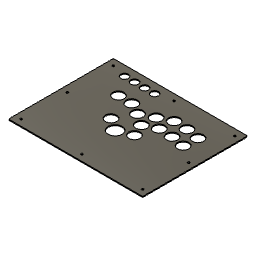
panel (Autodesk Fusion 360 design; units mm, degrees)
Autodesk Fusion 360 part; units mm, degrees
sketch "panel" plane through (0, 0, 0) normal (0, 0, 1) x (1, 0, 0)
  line L0 (62.8541, 263.5001) -> (357.1459, 263.5001)
  line L1 (357.1459, 263.5001) -> (357.1459, 33.5001)
  line L2 (357.1459, 33.5001) -> (62.8541, 33.5001)
  line L3 (62.8541, 33.5001) -> (62.8541, 263.5001)
  line L4 (137.8887, 199.6854) -> (139.7122, 197.8619)
  line L5 (139.7122, 199.6854) -> (137.8887, 197.8619)
  line L6 (167.3878, 199.4554) -> (169.2113, 197.6319)
  line L7 (169.2113, 199.4554) -> (167.3878, 197.6319)
  line L8 (193.5289, 185.7844) -> (195.3524, 183.9609)
  line L9 (195.3524, 185.7844) -> (193.5289, 183.9609)
  line L10 (220.9942, 199.2964) -> (222.8177, 197.4729)
  line L11 (222.8177, 199.2964) -> (220.9942, 197.4729)
  line L12 (247.5472, 212.1984) -> (249.3707, 210.3749)
  line L13 (249.3707, 212.1984) -> (247.5472, 210.3749)
  line L14 (277.0202, 210.8714) -> (278.8437, 209.0479)
  line L15 (278.8437, 210.8714) -> (277.0202, 209.0479)
  line L16 (306.1132, 205.9884) -> (307.9366, 204.1649)
  line L17 (307.9366, 205.9884) -> (306.1132, 204.1649)
  line L18 (304.0832, 175.4464) -> (305.9067, 173.6229)
  line L19 (305.9067, 175.4464) -> (304.0832, 173.6229)
  line L20 (274.9902, 180.3294) -> (276.8136, 178.5059)
  line L21 (276.8136, 180.3294) -> (274.9902, 178.5059)
  line L22 (245.5172, 181.6564) -> (247.3407, 179.8329)
  line L23 (247.3407, 181.6564) -> (245.5172, 179.8329)
  line L24 (218.9642, 168.7544) -> (220.7877, 166.9309)
  line L25 (220.7877, 168.7544) -> (218.9642, 166.9309)
  line L26 (230.8722, 141.9414) -> (232.6957, 140.1179)
  line L27 (232.6957, 141.9414) -> (230.8722, 140.1179)
  line L28 (173.1491, 148.1874) -> (174.9726, 146.3639)
  line L29 (174.9726, 148.1874) -> (173.1491, 146.3639)
  line L30 (200.3572, 129.9534) -> (202.1807, 128.1299)
  line L31 (202.1807, 129.9534) -> (200.3572, 128.1299)
  line L32 (108.0433, 242.9744) -> (109.8668, 241.1509)
  line L33 (109.8668, 242.9744) -> (108.0433, 241.1509)
  line L34 (130.0434, 242.9744) -> (131.8669, 241.1509)
  line L35 (131.8668, 242.9744) -> (130.0434, 241.1509)
  line L36 (152.0434, 242.9744) -> (153.8668, 241.1509)
  line L37 (153.8668, 242.9744) -> (152.0434, 241.1509)
  line L38 (174.0434, 242.9744) -> (175.8668, 241.1509)
  line L39 (175.8668, 242.9744) -> (174.0434, 241.1509)
  line L40 (75.8193, 250.5344) -> (77.6428, 248.7109)
  line L41 (77.6428, 250.5344) -> (75.8193, 248.7109)
  line L42 (75.8428, 149.3114) -> (77.6663, 147.4879)
  line L43 (77.6663, 149.3114) -> (75.8428, 147.4879)
  line L44 (75.8428, 48.1124) -> (77.6663, 46.2889)
  line L45 (77.6663, 48.1124) -> (75.8428, 46.2889)
  line L46 (209.1882, 250.5114) -> (211.0117, 248.6879)
  line L47 (211.0117, 250.5114) -> (209.1882, 248.6879)
  line L48 (342.5342, 149.3114) -> (344.3576, 147.4879)
  line L49 (344.3576, 149.3114) -> (342.5342, 147.4879)
  line L50 (342.5342, 250.5114) -> (344.3576, 248.6879)
  line L51 (344.3576, 250.5114) -> (342.5342, 248.6879)
  line L52 (342.5342, 48.1124) -> (344.3576, 46.2889)
  line L53 (344.3576, 48.1124) -> (342.5342, 46.2889)
  line L54 (209.1882, 48.1124) -> (211.0117, 46.2889)
  line L55 (211.0117, 48.1124) -> (209.1882, 46.2889)
  circle A0 centre (76.731, 249.6226) radius 2.3
  circle A1 centre (76.7545, 148.3996) radius 2.3
  circle A2 centre (76.7545, 47.2006) radius 2.3
  circle A3 centre (210.0999, 249.5996) radius 2.3
  circle A4 centre (343.4459, 249.5996) radius 2.3
  circle A5 centre (343.4459, 148.3996) radius 2.3
  circle A6 centre (343.4459, 47.2006) radius 2.3
  circle A7 centre (210.0999, 47.2006) radius 2.3
  circle A8 centre (138.8004, 198.7736) radius 12.3
  circle A9 centre (168.2995, 198.5436) radius 12.3
  circle A10 centre (194.4406, 184.8726) radius 12.3
  circle A11 centre (219.8759, 167.8426) radius 12.3
  circle A12 centre (221.9059, 198.3846) radius 12.3
  circle A13 centre (248.4589, 211.2866) radius 12.3
  circle A14 centre (246.4289, 180.7446) radius 12.3
  circle A15 centre (275.9019, 179.4176) radius 12.3
  circle A16 centre (277.9319, 209.9596) radius 12.3
  circle A17 centre (307.0249, 205.0766) radius 12.3
  circle A18 centre (304.9949, 174.5346) radius 12.3
  circle A19 centre (174.0608, 147.2756) radius 12.3
  circle A20 centre (231.7839, 141.0296) radius 12.3
  circle A21 centre (201.2689, 129.0416) radius 15.3
  circle A22 centre (108.9551, 242.0626) radius 8.3
  circle A23 centre (130.9551, 242.0626) radius 8.3
  circle A24 centre (152.9551, 242.0626) radius 8.3
  circle A25 centre (174.9551, 242.0626) radius 8.3
  dimension "d1" = 4.6
  dimension "d2" = 4.6
  dimension "d3" = 4.6
  dimension "d4" = 4.6
  dimension "d5" = 4.6
  dimension "d6" = 4.6
  dimension "d7" = 4.6
  dimension "d8" = 4.6
  dimension "d9" = 24.6
  dimension "d10" = 24.6
  dimension "d11" = 24.6
  dimension "d12" = 24.6
  dimension "d13" = 24.6
  dimension "d14" = 24.6
  dimension "d15" = 24.6
  dimension "d16" = 24.6
  dimension "d17" = 24.6
  dimension "d18" = 24.6
  dimension "d19" = 24.6
  dimension "d20" = 24.6
  dimension "d21" = 24.6
  dimension "d22" = 30.6
  dimension "d23" = 16.6
  dimension "d24" = 16.6
  dimension "d25" = 16.6
  dimension "d26" = 16.6
  constraint midpoint L41 A0.centre
  constraint midpoint L42 A1.centre
  constraint midpoint L45 A2.centre
  constraint midpoint L46 A3.centre
  constraint midpoint L50 A4.centre
  constraint midpoint L48 A5.centre
  constraint midpoint L53 A6.centre
  constraint midpoint L54 A7.centre
  constraint midpoint L5 A8.centre
  constraint midpoint L7 A9.centre
  constraint midpoint L8 A10.centre
  constraint midpoint L24 A11.centre
  constraint midpoint L11 A12.centre
  constraint midpoint L12 A13.centre
  constraint midpoint L23 A14.centre
  constraint midpoint L20 A15.centre
  constraint midpoint L15 A16.centre
  constraint midpoint L16 A17.centre
  constraint midpoint L19 A18.centre
  constraint midpoint L29 A19.centre
  constraint midpoint L27 A20.centre
  constraint midpoint L31 A21.centre
  constraint midpoint L33 A22.centre
  constraint midpoint L34 A23.centre
  constraint midpoint L36 A24.centre
  constraint midpoint L39 A25.centre
  measures "d1" diameter of A0
  measures "d2" diameter of A1
  measures "d3" diameter of A2
  measures "d4" diameter of A3
  measures "d5" diameter of A4
  measures "d6" diameter of A5
  measures "d7" diameter of A6
  measures "d8" diameter of A7
  measures "d9" diameter of A8
  measures "d10" diameter of A9
  measures "d11" diameter of A10
  measures "d12" diameter of A11
  measures "d13" diameter of A12
  measures "d14" diameter of A13
  measures "d15" diameter of A14
  measures "d16" diameter of A15
  measures "d17" diameter of A16
  measures "d18" diameter of A17
  measures "d19" diameter of A18
  measures "d20" diameter of A19
  measures "d21" diameter of A20
  measures "d22" diameter of A21
  measures "d23" diameter of A22
  measures "d24" diameter of A23
  measures "d25" diameter of A24
  measures "d26" diameter of A25
extrude "Extrude1" add sketch "panel" along normal blind 2
fillet "Fillet1" radius 2 4 edges at (62.8541, 33.5001, 1) (62.8541, 263.5001, 1) (357.1459, 33.5001, 1) (357.1459, 263.5001, 1)
